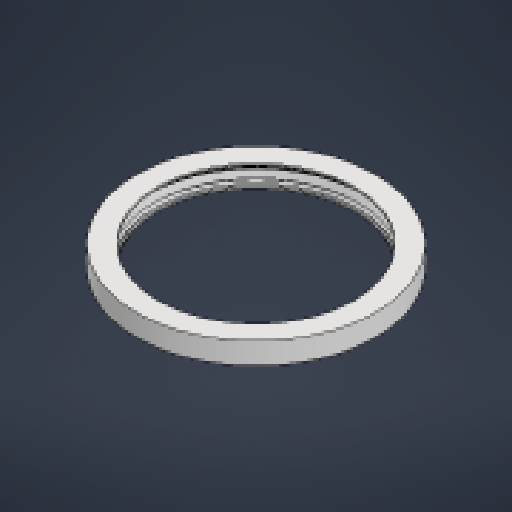
# Autodesk Inventor part: 3DPRINT,OUTER-V
Saved by Autodesk Inventor 2026 (Build 300175000, 175)
## iProperties
Created: 2026-02-03
Part Number: 3DPRINT,OUTER-V
Material: Nylon 6/6
Document SubType Name: Modeling
Designer: littl
Density: 1.13 g/cm^3
Appearance: Nylon 6
Author: littl
Autodesk Inventor part; units mm, degrees
ref_plane "YZ Plane" through (0, 0, 0) normal (1, 0, 0) x (0, 1, 0)
ref_plane "XZ Plane" through (0, 0, 0) normal (0, 1, 0) x (-1, 0, 0)
ref_plane "XY Plane" through (0, 0, 0) normal (0, 0, 1) x (1, 0, 0)
sketch "Sketch1" plane through (0, 0, 0) normal (0, 0, 1) x (1, 0, 0)
  line L0 (0, -12.446) -> (0, 12.446) projected
  line L1 (-129.54, 0) -> (21.59, 0) construction
  line L2 (-107.95, 8.89) -> (-107.95, 0)
  line L3 (-107.95, 8.89) -> (-90.3815, 8.89)
  line L4 (-90.3815, 8.89) -> (-90.3815, 7.3025)
  line L5 (-90.3815, 7.3025) -> (-91.504, 6.18)
  line L6 (-91.504, 6.18) -> (-92.9409, 7.6168)
  line L7 (-92.9409, 7.6168) -> (-95.186, 5.3717)
  line L8 (-95.186, 5.3717) -> (-93.7491, 3.9349)
  line L9 (-93.7491, 3.9349) -> (-97.684, 0)
  line L10 (-97.176, 0) -> (-88.9855, 8.1905) construction
  line L11 (-94.0634, 6.4943) -> (-92.3726, 4.8034) construction
  circle A0 centre (-93.218, 5.6489) radius 1.3081 construction
  line L12 (-107.95, -8.89) -> (-90.3815, -8.89) construction
  line L13 (-90.3815, -8.89) -> (-90.3815, -7.3025) construction
  line L14 (-90.3815, -7.3025) -> (-91.504, -6.18) construction
  line L15 (-91.504, -6.18) -> (-92.9409, -7.6168) construction
  line L16 (-92.9409, -7.6168) -> (-95.186, -5.3717) construction
  line L17 (-95.186, -5.3717) -> (-93.7491, -3.9349) construction
  line L18 (-93.7491, -3.9349) -> (-97.684, 0) construction
  line L19 (-107.95, 0) -> (-97.684, 0)
  line L20 (-107.95, 0) -> (-107.95, -8.89) construction
  point P0 (0, 0)
  dimension "d24" = 1.5875
  dimension "d25" = 2.032
  dimension "d26" = 45
  dimension "d27" = 0.508
  dimension "d28" = 3.175
  dimension "d29" = 2.6162
  dimension "d30" = 186.436
  dimension "d31" = 215.9
  dimension "d32" = 17.78
  dimension "d33" = 1.5875
  constraints: 38 end point, 7 point on line, 7 symmetric about line, 5 perpendicular, 2 horizontal, 2 midpoint, 2 vertical, 1 centre point, 1 parallel
  measures "d24" distance of L3.end L4.end
  measures "d25" distance of L5.end L6.end
  measures "d26" angle of L1 L9
  measures "d27" distance of L10.start L9.end
  measures "d28" distance of L6.end L7.end
  measures "d29" diameter of A0
  measures "d30" diameter of A0.centre L0
  measures "d31" diameter of L2 L0
  measures "d32" distance of L2.start L12.start
  measures "d33" distance of L4.end L5.end
revolve "Revolution1" add sketch "Sketch1" angle 360 about axis through (0, -10, 0) along (0, 1, 0)
sketch "Sketch2" plane through (0, 8.89, 0) normal (0, 1, 0) x (1, 0, 0)
  point P0 (0, 0)
  point P1 (0, 102.87)
  point P2 (-89.088, 51.435)
  point P3 (-89.088, -51.435)
  point P4 (0, -102.87)
  point P5 (89.088, -51.435)
  point P6 (89.088, 51.435)
  dimension "d36" = 102.87
  dimension "d39" = 360
  constraints: 1 vertical alignment, 7 other
  measures "d36" distance of point (0, 0) point (0, 102.87)
hole "Hole1" at (0, 8.89, -102.87) at (-89.088, 8.89, -51.435) at (-89.088, 8.89, 51.435) at (0, 8.89, 102.87) at (89.088, 8.89, 51.435) at (89.088, 8.89, -51.435) direction (0, -1, 0) diameter 5.1054 end through all clearance for "Flat Head Machine Screw (82)" size "#10" standard "Ansi Unified Screw Threads"
body "Solid1"
